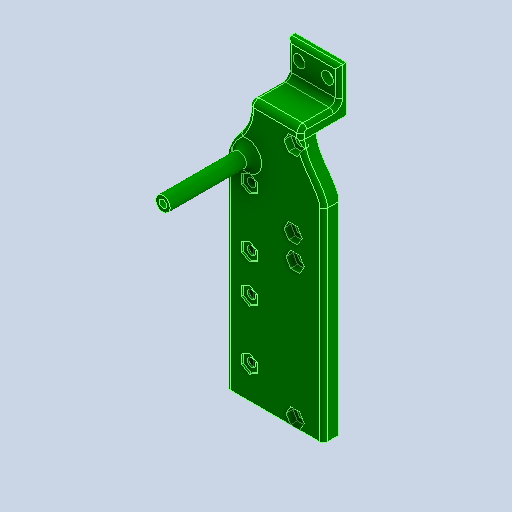
# Autodesk Inventor part: Battery_holder
Saved by Autodesk Inventor 2023.1 (Build 271208000, 208)
## iProperties
Created: 2022-08-12
Part Number: Battery_holder
Material: Default New Material
Document SubType Name: Modeling
Designer: Windows10
Density: 1 g/cm^3
Appearance: Generic
Author: Windows10
Autodesk Inventor part; units mm, degrees
ref_plane "YZ Plane" through (0, 0, 0) normal (1, 0, 0) x (0, 1, 0)
ref_plane "XZ Plane" through (0, 0, 0) normal (0, 1, 0) x (-1, 0, 0)
ref_plane "XY Plane" through (0, 0, 0) normal (0, 0, 1) x (1, 0, 0)
ref_plane "Work Plane2" through (3.3864, -46.8933, 3) normal (0, 0, 1) x (1, 0, 0)
sketch "Sketch1" plane through (3.3864, -46.8933, 3) normal (0, 0, 1) x (1, 0, 0)
  line L0 (-6.3864, -93.5067) -> (19.0636, -93.5067)
  line L1 (19.0636, -93.5067) -> (19.0636, -105.5067)
  line L2 (19.0636, -105.5067) -> (-6.3864, -105.5067)
  line L3 (-6.3864, -105.5067) -> (-6.3864, -93.5067)
  line L4 (-0.3864, -19.9067) -> (-0.3864, -27.9067) projected
  line L5 (-0.3864, -27.9067) -> (13.0636, -27.9067) projected
  line L6 (13.0636, -27.9067) -> (13.0636, -19.9067) projected
  line L7 (-0.3864, -27.9067) -> (-0.3864, -22.9067) projected
  line L8 (-0.3864, -27.9067) -> (13.0636, -27.9067)
  line L9 (13.0636, -27.9067) -> (13.0636, -15.9067)
  line L10 (13.0636, -15.9067) -> (-0.3864, -15.9067)
  line L11 (-0.3864, -15.9067) -> (-0.3864, -27.9067)
  point P0 (-3.3864, 46.8933)
  dimension "d1" = 25.45
  dimension "d2" = 12
  dimension "d3" = 13.45
  dimension "d4" = 12
  constraints: 16 end point, 4 parallel, 2 horizontal, 2 perpendicular
  measures "d1" distance of L1.end L2.end
  measures "d2" distance of L0.end L1.end
  measures "d3" distance of L10.end L9.end
  measures "d4" distance of L10.end L4.end
extrude "Extrusion1" add sketch "Sketch1" along normal blind 2
ref_plane "Work Plane3" through (3.3864, -46.8933, 5) normal (0, 0, 1) x (1, 0, 0)
sketch "Sketch2" plane through (3.3864, -46.8933, 5) normal (0, 0, 1) x (1, 0, 0)
  line L0 (19.0636, -93.5067) -> (-6.3864, -93.5067) projected
  line L1 (19.0636, -105.5067) -> (19.0636, -93.5067) projected
  line L2 (-6.3864, -93.5067) -> (19.0636, -93.5067)
  line L3 (19.0636, -93.5067) -> (19.0636, -96.5067)
  line L4 (19.0636, -96.5067) -> (-6.3864, -96.5067)
  line L5 (-6.3864, -96.5067) -> (-6.3864, -93.5067)
  line L6 (-0.3864, -27.9067) -> (-0.3864, -22.9067) projected
  line L7 (13.0636, -22.9067) -> (13.0636, -27.9067) projected
  line L8 (-0.3864, -27.9067) -> (13.0636, -27.9067)
  line L9 (13.0636, -27.9067) -> (13.0636, -24.9067)
  line L10 (13.0636, -24.9067) -> (-0.3864, -24.9067)
  line L11 (-0.3864, -24.9067) -> (-0.3864, -27.9067)
  point P0 (-3.3864, 46.8933)
  point P1 (-0.3864, -24.9067)
  dimension "d7" = 3
  dimension "d8" = 3
  constraints: 16 end point, 4 parallel, 2 horizontal, 2 perpendicular, 2 point on line
  measures "d7" distance of L2.end L3.end
  measures "d8" distance of L9.end L8.end
extrude "Extrusion2" add sketch "Sketch2" along normal blind 6
sketch "Sketch3" plane through (3.3864, -46.8933, 11) normal (0, 0, 1) x (1, 0, 0)
  line L0 (-6.3864, -96.5067) -> (19.0636, -96.5067) projected
  line L1 (19.0636, -96.5067) -> (19.0636, -93.5067) projected
  line L2 (19.0636, -93.5067) -> (-6.3864, -93.5067) projected
  line L3 (-6.3864, -93.5067) -> (-6.3864, -96.5067) projected
  line L4 (13.0636, -27.9067) -> (13.0636, -24.9067) projected
  line L5 (13.0636, -24.9067) -> (-0.3864, -24.9067) projected
  line L6 (-0.3864, -24.9067) -> (-0.3864, -27.9067) projected
  line L7 (-0.3864, -27.9067) -> (13.0636, -27.9067) projected
  line L8 (-6.3864, -96.5067) -> (19.0636, -96.5067)
  line L9 (19.0636, -96.5067) -> (19.0636, -40.4712)
  line L10 (19.0636, -40.4712) -> (-6.3864, -40.4712)
  line L11 (-6.3864, -40.4712) -> (-6.3864, -96.5067)
  line L12 (-6.3864, -40.4712) -> (-6.3864, -37.4338) construction
  line L13 (-6.3864, -37.4338) -> (-3.3864, -34.2758) construction
  line L14 (-3.3864, -34.2758) -> (-1.0738, -32.4773) construction
  line L15 (-1.0738, -32.4773) -> (-0.3864, -27.9067) construction
  spline S0 degree 4 poles (-6.3864, -40.4712) (-6.3864, -37.4338) (-3.3864, -34.2758) (-1.0738, -32.4773) (-0.3864, -27.9067) knots 1 1 1 1 1 2 2 2 2 2
  line L16 (6.3386, -40.4712) -> (6.3386, -46.7803)
  line L17 (19.0636, -40.4712) -> (19.0636, -37.4338) construction
  line L18 (19.0636, -37.4338) -> (16.0636, -34.2758) construction
  line L19 (16.0636, -34.2758) -> (13.7511, -32.4773) construction
  line L20 (13.7511, -32.4773) -> (13.0636, -27.9067) construction
  spline S1 degree 4 poles (19.0636, -40.4712) (19.0636, -37.4338) (16.0636, -34.2758) (13.7511, -32.4773) (13.0636, -27.9067) knots 1 1 1 1 1 2 2 2 2 2
  point P0 (-3.3864, 46.8933)
  point P1 (-6.3864, -93.5067)
  dimension "d11" = 25.45
  constraints: 10 end point, 3 symmetric about line, 2 parallel, 2 vertical, 1 horizontal, 1 midpoint, 1 perpendicular, 6 other
  measures "d11" distance of L10.end L9.end
extrude "Extrusion3" add sketch "Sketch3" along normal blind 4
sketch "Sketch4" plane through (3.3864, -46.8933, 5) normal (0, 0, 1) x (1, 0, 0)
  circle A0 centre (-1.3864, -101.5067) radius 1.75
  line L0 (-6.3864, -105.5067) -> (19.0636, -105.5067) projected
  line L1 (6.3386, -105.5067) -> (6.3386, -103.8916)
  line L2 (-6.3864, -96.5067) -> (-6.3864, -105.5067) projected
  line L3 (-6.3864, -96.5067) -> (19.0636, -96.5067) projected
  circle A1 centre (14.0636, -101.5067) radius 1.75
  circle A2 centre (2.6136, -19.9067) radius 1.5475
  line L4 (13.0636, -15.9067) -> (-0.3864, -15.9067) projected
  line L5 (6.3386, -15.9067) -> (6.3386, -14.3584)
  line L6 (-0.3864, -15.9067) -> (-0.3864, -24.9067) projected
  circle A3 centre (10.0636, -19.9067) radius 1.5475
  line L7 (13.0636, -24.9067) -> (-0.3864, -24.9067) projected
  point P0 (-3.3864, 46.8933)
  point P1 (-6.3864, -98.0067)
  dimension "d15" = 3.5
  dimension "d16" = 5
  dimension "d17" = 4
  dimension "d18" = 3
  dimension "d19" = 4
  dimension "d23" = 5
  dimension "d24" = 5
  dimension "d89" = 81.6
  dimension "d90" = 4
  dimension "d91" = 7.45
  dimension "d92" = 15.45
  dimension "d93" = 4
  constraints: 4 centre point, 4 end point, 2 midpoint, 2 symmetric about line, 2 vertical, 2 other
  measures "d15" diameter of A0
  measures "d16" distance from line of A0.centre L2
  measures "d17" distance from line of L0 A0.centre
  measures "d18" distance from line of L6 A2.centre
  measures "d19" distance from line of L4 A2.centre
  measures "d23" distance from line of L3 A0.centre
  measures "d24" distance from line of A2.centre L7
  measures "d89" vertical distance of A1.centre A3.centre
  measures "d90" horizontal distance of A3.centre A1.centre
  measures "d91" distance of A2.centre A3.centre
  measures "d92" distance of A0.centre A1.centre
  measures "d93" horizontal distance of A2.centre A0.centre
extrude "Extrusion4" cut sketch "Sketch4" against normal blind 2
fillet "Fillet2" radius 1.5 4 edges at (9.725, -143.4, 15) (9.725, -143.4, 5) (9.725, -71.8, 15) (9.725, -71.8, 5)
sketch "Sketch6" plane through (3.3864, -46.8933, 15) normal (0, 0, 1) x (1, 0, 0)
  line L0 (9.0398, -52.206) -> (21.0398, -52.206)
  line L1 (21.0398, -52.206) -> (21.0398, -27.206)
  line L2 (21.0398, -27.206) -> (9.0398, -27.206)
  line L3 (9.0398, -27.206) -> (9.0398, -52.206)
  line L4 (9.0398, -93.9784) -> (29.3398, -93.9784)
  line L5 (29.3398, -93.9784) -> (29.3398, -53.3784)
  line L6 (29.3398, -53.3784) -> (9.0398, -53.3784)
  line L7 (9.0398, -53.3784) -> (9.0398, -93.9784)
  circle A0 centre (11.0398, -29.706) radius 1.1
  circle A1 centre (11.5798, -91.4384) radius 1.1
  line L8 (9.0398, -73.6784) -> (6.4211, -73.6784)
  circle A2 centre (11.5798, -55.9184) radius 1.1
  line L9 (12.7648, -89.3859) -> (13.9498, -91.4384)
  line L10 (13.9498, -91.4384) -> (12.7648, -93.4909)
  line L11 (12.7648, -93.4909) -> (10.3948, -93.4909)
  line L12 (10.3948, -93.4909) -> (9.2098, -91.4384)
  line L13 (9.2098, -91.4384) -> (10.3948, -89.3859)
  line L14 (10.3948, -89.3859) -> (12.7648, -89.3859)
  circle A3 centre (11.5798, -91.4384) radius 3.5
  circle A4 centre (11.5798, -55.9184) radius 1.1
  line L15 (12.7648, -57.9709) -> (13.9498, -55.9184)
  line L16 (13.9498, -55.9184) -> (12.7648, -53.8659)
  line L17 (12.7648, -53.8659) -> (10.3948, -53.8659)
  line L18 (10.3948, -53.8659) -> (9.2098, -55.9184)
  line L19 (9.2098, -55.9184) -> (10.3948, -57.9709)
  line L20 (10.3948, -57.9709) -> (12.7648, -57.9709)
  circle A5 centre (11.5798, -55.9184) radius 3.5
  circle A6 centre (11.0398, -29.706) radius 1.1
  line L21 (9.8548, -31.7585) -> (12.2248, -31.7585)
  line L22 (8.6698, -29.706) -> (9.8548, -31.7585)
  line L23 (12.2248, -31.7585) -> (13.4098, -29.706)
  circle A7 centre (11.0398, -29.706) radius 1.1
  line L24 (13.4098, -29.706) -> (12.2248, -27.6536)
  line L25 (12.2248, -27.6536) -> (9.8548, -27.6536)
  line L26 (9.8548, -27.6536) -> (8.6698, -29.706)
  circle A8 centre (11.0398, -29.706) radius 3.5
  line L27 (-0.3864, -26.4067) -> (13.0636, -26.4067) projected
  line L28 (6.3386, -26.4067) -> (6.3386, -33.206)
  line L29 (3.6375, -27.206) -> (3.6375, -52.206)
  circle A9 centre (1.6375, -29.706) radius 1.1
  line L30 (4.0075, -29.706) -> (2.8225, -31.7585)
  line L31 (2.8225, -31.7585) -> (0.4525, -31.7585)
  line L32 (0.4525, -27.6536) -> (2.8225, -27.6536)
  line L33 (-0.7325, -29.706) -> (0.4525, -27.6536)
  line L34 (2.8225, -27.6536) -> (4.0075, -29.706)
  line L35 (0.4525, -31.7585) -> (-0.7325, -29.706)
  line L36 (13.0636, -23.4067) -> (-0.3864, -23.4067) projected
  line L37 (9.0398, -39.706) -> (7.6363, -39.706)
  circle A10 centre (11.0398, -49.706) radius 1.1
  line L38 (8.6698, -49.706) -> (9.8548, -47.6536)
  line L39 (9.8548, -47.6536) -> (12.2248, -47.6536)
  line L40 (12.2248, -51.7585) -> (9.8548, -51.7585)
  line L41 (13.4098, -49.706) -> (12.2248, -51.7585)
  line L42 (9.8548, -51.7585) -> (8.6698, -49.706)
  line L43 (12.2248, -47.6536) -> (13.4098, -49.706)
  circle A11 centre (-0.3864, -85.0067) radius 1.1
  line L44 (-6.3864, -40.4712) -> (-6.3864, -95.0067) projected
  line L45 (-0.3864, -85.0067) -> (-0.3864, -77.2817)
  line L46 (-0.3864, -77.2817) -> (0.7136, -77.2817)
  line L47 (-0.3864, -87.3767) -> (-2.4389, -86.1917)
  line L48 (-2.4389, -86.1917) -> (-2.4389, -83.8217)
  line L49 (-2.4389, -83.8217) -> (-0.3864, -82.6366)
  line L50 (-0.3864, -82.6366) -> (1.6661, -83.8217)
  line L51 (1.6661, -83.8217) -> (1.6661, -86.1917)
  line L52 (1.6661, -86.1917) -> (-0.3864, -87.3767)
  circle A12 centre (-0.3864, -69.5567) radius 1.1
  line L53 (-0.3864, -67.1866) -> (-2.4389, -68.3717)
  line L54 (-2.4389, -68.3717) -> (-2.4389, -70.7417)
  line L55 (-2.4389, -70.7417) -> (-0.3864, -71.9267)
  line L56 (-0.3864, -71.9267) -> (1.6661, -70.7417)
  line L57 (1.6661, -70.7417) -> (1.6661, -68.3717)
  line L58 (1.6661, -68.3717) -> (-0.3864, -67.1866)
  line L59 (9.0398, -64.5567) -> (-9.8125, -64.5567)
  circle A13 centre (-0.3864, -44.1067) radius 1.1
  line L60 (-0.3864, -44.1067) -> (-0.3864, -51.8317)
  line L61 (-0.3864, -51.8317) -> (0.7136, -51.8317)
  line L62 (-0.3864, -41.7366) -> (-2.4389, -42.9217)
  line L63 (-2.4389, -42.9217) -> (-2.4389, -45.2917)
  line L64 (-2.4389, -45.2917) -> (-0.3864, -46.4767)
  line L65 (-0.3864, -46.4767) -> (1.6661, -45.2917)
  line L66 (1.6661, -45.2917) -> (1.6661, -42.9217)
  line L67 (1.6661, -42.9217) -> (-0.3864, -41.7366)
  line L68 (-2.4389, -60.7417) -> (-2.4389, -58.3717)
  circle A14 centre (-0.3864, -59.5567) radius 1.1
  line L69 (-0.3864, -57.1866) -> (1.6661, -58.3717)
  line L70 (1.6661, -58.3717) -> (1.6661, -60.7417)
  line L71 (1.6661, -60.7417) -> (-0.3864, -61.9267)
  line L72 (-0.3864, -61.9267) -> (-2.4389, -60.7417)
  line L73 (-2.4389, -58.3717) -> (-0.3864, -57.1866)
  line L74 (-3.4389, -83.2443) -> (-3.4389, -86.769)
  line L75 (-3.4389, -86.769) -> (-0.3864, -88.5314)
  line L76 (-0.3864, -88.5314) -> (2.6661, -86.769)
  line L77 (2.6661, -86.769) -> (2.6661, -83.2443)
  line L78 (2.6661, -83.2443) -> (-0.3864, -81.4819)
  line L79 (-0.3864, -81.4819) -> (-3.4389, -83.2443)
  line L80 (-3.4389, -71.319) -> (-3.4389, -67.7943)
  line L81 (-3.4389, -67.7943) -> (-0.3864, -66.0319)
  line L82 (-0.3864, -66.0319) -> (2.6661, -67.7943)
  line L83 (2.6661, -67.7943) -> (2.6661, -71.319)
  line L84 (2.6661, -71.319) -> (-0.3864, -73.0814)
  line L85 (-0.3864, -73.0814) -> (-3.4389, -71.319)
  line L86 (-3.4389, -57.7943) -> (-3.4389, -61.319)
  line L87 (-3.4389, -61.319) -> (-0.3864, -63.0814)
  line L88 (-0.3864, -63.0814) -> (2.6661, -61.319)
  line L89 (2.6661, -61.319) -> (2.6661, -57.7943)
  line L90 (2.6661, -57.7943) -> (-0.3864, -56.0319)
  line L91 (-0.3864, -56.0319) -> (-3.4389, -57.7943)
  line L92 (-3.4389, -42.3443) -> (-0.3864, -40.5819)
  line L93 (-0.3864, -40.5819) -> (2.6661, -42.3443)
  line L94 (2.6661, -42.3443) -> (2.6661, -45.869)
  line L95 (2.6661, -45.869) -> (-0.3864, -47.6314)
  line L96 (-0.3864, -47.6314) -> (-3.4389, -45.869)
  line L97 (-3.4389, -45.869) -> (-3.4389, -42.3443)
  point P0 (-3.3864, 46.8933)
  point P1 (15.0398, -52.206)
  point P2 (8.4998, -46.166)
  point P3 (8.4998, -27.166)
  point P4 (-6.3864, -96.5067)
  point P5 (-0.3864, -64.5567)
  point P6 (6.4211, -55.4349)
  dimension "d47" = 12
  dimension "d48" = 25
  dimension "d49" = 20.3
  dimension "d50" = 40.6
  dimension "d54" = 2.2
  dimension "d55" = 2
  dimension "d56" = 2.5
  dimension "d57" = 2.2
  dimension "d58" = 2.54
  dimension "d59" = 2.54
  dimension "d60" = 4.74
  dimension "d61" = 7
  dimension "d99" = 4.2469
  dimension "d100" = 2.54
  dimension "d101" = 2.2
  dimension "d102" = 6
  dimension "d103" = 4.105
  dimension "d104" = 11.5
  dimension "d105" = 7.725
  dimension "d106" = 4.105
  dimension "d107" = 5
  dimension "d108" = 1
  dimension "d109" = 1
  dimension "d110" = 1
  dimension "d111" = 1
  constraints: 190 end point, 53 symmetric about line, 15 centre point, 7 coincident, 6 horizontal, 5 midpoint, 4 parallel, 2 perpendicular, 2 vertical, 1 collinear, 1 point on line, 54 other
  measures "d47" distance of L2.end L1.end
  measures "d48" distance of L1.end L0.end
  measures "d49" distance of L6.end L5.end
  measures "d50" distance of L5.end L4.end
  measures "d54" diameter of A0
  measures "d55" distance from line of A0.centre L3
  measures "d56" distance from line of L2 A0.centre
  measures "d57" diameter of A1
  measures "d58" distance from line of L7 A1.centre
  measures "d59" distance from line of L4 A1.centre
  measures "d60" distance of L9.end L12.end
  measures "d61" diameter of A3
  measures "d99" distance between parallel lines of L36 L25
  measures "d100" distance from line of L7 A5.centre
  measures "d101" diameter of A11
  measures "d102" distance from line of L44 L45.start
  measures "d103" distance between parallel lines of L14 L11
  measures "d104" vertical distance of point (-6.386, -96.507) L45.start
  measures "d105" distance of L45.start L45.end
  measures "d106" distance between parallel lines of L51 L48
  measures "d107" distance of A12.centre point (-0.386, -64.557)
  measures "d108" distance between parallel lines of L48 L74
  measures "d109" distance between parallel lines of L54 L80
  measures "d110" distance between parallel lines of L68 L86
  measures "d111" distance between parallel lines of L62 L92
extrude "Extrusion5" cut sketch "Sketch6" against normal blind 1.8 contours L42 L38 L3 | L3 L38 L39 L43 L41 L40 L42 | L26 L25 L24 L23 L21 L22 L3 | L3 L22 L26 | A0 | A1 | A2 | L9 L10 L11 L12 L13 L14 | L20 L19 L18 L17 L16 L15 | A10
ref_plane "Work Plane4" through (-3, -140.4, 3) normal (0, 1, 0) x (1, 0, 0)
split body "Split1" result two bodies by plane through (-3, -140.4, 3) normal (0, 1, 0) first body at (13.9667, -122.7215, 11.5)
sketch "Sketch7" plane through (-3, -140.4, 15) normal (0, -1, 0) x (1, 0, 0)
  line L0 (14.45, -1) -> (4, -1)
  line L1 (4, -1) -> (4, -3)
  line L2 (4, -3) -> (14.45, -3)
  line L3 (14.45, -3) -> (14.45, -1)
  line L4 (25.45, -4) -> (25.45, 0) projected
  line L5 (0, 0) -> (0, -4) projected
  line L6 (25.45, -4) -> (0, -4) projected
  line L7 (25.45, 0) -> (0, 0) projected
  point P0 (3, -15)
  point P1 (15.5961, 0)
  point P2 (25.45, -2)
  dimension "d65" = 11
  dimension "d66" = 4
  dimension "d67" = 2
  dimension "d69" = 1
  dimension "d70" = 1
  constraints: 8 end point, 2 parallel, 1 horizontal, 1 midpoint, 1 perpendicular
  measures "d65" distance from line of point (25.45, -2) L3
  measures "d66" distance between parallel lines of L5 L1
  measures "d67" distance of L0.end L1.end
  measures "d69" distance between parallel lines of L7 L0
  measures "d70" distance between parallel lines of L6 L2
extrude "Extrusion6" cut sketch "Sketch7" against normal blind 48 contours L3 L2 L1 L0 bodies 2
sketch "Sketch8" plane through (-3, -140.4, 3) normal (0, 1, 0) x (1, 0, 0)
  line L0 (14.45, -1.1) -> (4, -1.1)
  line L1 (4, -1.1) -> (4, -2.9)
  line L2 (4, -2.9) -> (14.45, -2.9)
  line L3 (14.45, -2.9) -> (14.45, -1.1)
  line L4 (25.45, -4) -> (25.45, 0)
  line L5 (0, 0) -> (0, -4)
  line L6 (25.45, -4) -> (0, -4)
  line L7 (25.45, 0) -> (0, 0)
  line L8 (30.2309, -12) -> (30.2309, 0)
  line L9 (30.2309, -6) -> (31.8513, -6)
  line L10 (14.45, -10.9) -> (4, -10.9)
  line L11 (4, -10.9) -> (4, -9.1)
  line L12 (4, -9.1) -> (14.45, -9.1)
  line L13 (14.45, -9.1) -> (14.45, -10.9)
  line L14 (25.45, -8) -> (25.45, -12)
  line L15 (0, -12) -> (0, -8)
  line L16 (25.45, -8) -> (0, -8)
  line L17 (25.45, -12) -> (0, -12)
  line L18 (4.3, -10.6) -> (14.15, -10.6)
  line L19 (14.15, -10.6) -> (14.15, -9.4)
  line L20 (14.15, -9.4) -> (4.3, -9.4)
  line L21 (4.3, -9.4) -> (4.3, -10.6)
  point P0 (3, 3)
  point P1 (3, -15)
  point P2 (15.5961, 0)
  point P3 (25.45, -2)
  point P4 (15.5961, -12)
  point P5 (25.45, -10)
  dimension "d73" = 11
  dimension "d74" = 4
  dimension "d75" = 1.8
  dimension "d76" = 1.1
  dimension "d77" = 1.1
  dimension "d78" = 0.3
  constraints: 44 end point, 10 symmetric about line, 2 horizontal, 2 midpoint, 2 parallel, 1 perpendicular, 1 vertical, 3 other
  measures "d73" distance from line of point (25.45, -2) L3
  measures "d74" distance between parallel lines of L5 L1
  measures "d75" distance of L0.end L1.end
  measures "d76" distance between parallel lines of L7 L0
  measures "d77" distance between parallel lines of L6 L2
  measures "d78" distance between parallel lines of L10 L18
extrude "Extrusion7" add sketch "Sketch8" along normal blind 48 contours L21 L20 L19 L18 bodies 3
sketch "Sketch9" plane through (3.3864, -46.8933, 15) normal (0, 0, 1) x (1, 0, 0)
  line L0 (-1.0605, -90.0613) -> (-1.0605, -38.0613)
  circle A0 centre (-1.0605, -90.0613) radius 1
  circle A1 centre (-1.0605, -38.0613) radius 1
  circle A2 centre (-1.0605, -90.0613) radius 1.9
  circle A3 centre (-1.0605, -38.0613) radius 1.9
  line L1 (19.0636, -93.5067) -> (-6.3864, -93.5067) projected
  point P0 (-3.3864, 46.8933)
  point P1 (-3.3864, 46.8933)
  dimension "d81" = 52
  dimension "d82" = 2
  dimension "d83" = 2
  dimension "d84" = 3.8
  dimension "d85" = 3.8
  dimension "d150" = 3.4453
  constraints: 4 centre point, 4 coincident, 2 end point, 1 vertical
  measures "d81" distance of L0.start L0.end
  measures "d82" diameter of A0
  measures "d83" diameter of A1
  measures "d84" diameter of A2
  measures "d85" diameter of A3
  measures "d150" distance from line of L1 L0.start
extrude "Extrusion8" add sketch "Sketch9" along normal blind 22 contours A3 bodies 2
fillet "Fillet3" radius 2 1 edges at (0.4258, -84.9547, 15)
extrude "Extrusion9" cut sketch "Sketch6" against normal blind 12.25 contours A0 | A1 | A2 | A10 bodies 2
extrude "Extrusion10" [suppressed]
sketch "Sketch11" plane through (3.3864, -46.8933, 16.5) normal (0, 0, 1) x (1, 0, 0)
  line L0 (9.0398, -52.206) -> (21.0398, -52.206)
  line L1 (21.0398, -52.206) -> (21.0398, -27.206)
  line L2 (21.0398, -27.206) -> (9.0398, -27.206)
  line L3 (9.0398, -27.206) -> (9.0398, -52.206)
  line L4 (9.0398, -93.9784) -> (29.3398, -93.9784)
  line L5 (29.3398, -93.9784) -> (29.3398, -53.3784)
  line L6 (29.3398, -53.3784) -> (9.0398, -53.3784)
  line L7 (9.0398, -53.3784) -> (9.0398, -93.9784)
  circle A0 centre (11.0398, -29.706) radius 1.1
  circle A1 centre (11.5798, -91.4384) radius 1.1
  line L8 (9.0398, -73.6784) -> (6.4211, -73.6784)
  circle A2 centre (11.5798, -55.9184) radius 1.1
  line L9 (12.7648, -89.3859) -> (13.9498, -91.4384)
  line L10 (13.9498, -91.4384) -> (12.7648, -93.4909)
  line L11 (12.7648, -93.4909) -> (10.3948, -93.4909)
  line L12 (10.3948, -93.4909) -> (9.2098, -91.4384)
  line L13 (9.2098, -91.4384) -> (10.3948, -89.3859)
  line L14 (10.3948, -89.3859) -> (12.7648, -89.3859)
  circle A3 centre (11.5798, -91.4384) radius 3.5
  line L15 (10.3948, -57.9709) -> (12.7648, -57.9709)
  line L16 (9.2098, -55.9184) -> (10.3948, -57.9709)
  line L17 (12.7648, -57.9709) -> (13.9498, -55.9184)
  circle A4 centre (11.5798, -55.9184) radius 1.1
  line L18 (13.9498, -55.9184) -> (12.7648, -53.8659)
  line L19 (12.7648, -53.8659) -> (10.3948, -53.8659)
  line L20 (10.3948, -53.8659) -> (9.2098, -55.9184)
  circle A5 centre (11.5798, -55.9184) radius 3.5
  line L21 (8.6698, -29.706) -> (9.8548, -31.7585)
  line L22 (9.8548, -31.7585) -> (12.2248, -31.7585)
  circle A6 centre (11.0398, -29.706) radius 3.5
  circle A7 centre (11.0398, -29.706) radius 1.1
  line L23 (12.2248, -27.6536) -> (9.8548, -27.6536)
  line L24 (13.4098, -29.706) -> (12.2248, -27.6536)
  line L25 (9.8548, -27.6536) -> (8.6698, -29.706)
  circle A8 centre (11.0398, -29.706) radius 1.1
  line L26 (12.2248, -31.7585) -> (13.4098, -29.706)
  line L27 (-0.3864, -26.4067) -> (13.0636, -26.4067)
  line L28 (6.3386, -26.4067) -> (6.3386, -33.206)
  line L29 (4.0075, -29.706) -> (2.8225, -31.7585)
  line L30 (3.6375, -27.206) -> (3.6375, -52.206)
  line L31 (0.4525, -27.6536) -> (2.8225, -27.6536)
  line L32 (-0.7325, -29.706) -> (0.4525, -27.6536)
  line L33 (0.4525, -31.7585) -> (-0.7325, -29.706)
  line L34 (2.8225, -31.7585) -> (0.4525, -31.7585)
  circle A9 centre (1.6375, -29.706) radius 1.1
  line L35 (2.8225, -27.6536) -> (4.0075, -29.706)
  line L36 (13.0636, -23.4067) -> (-0.3864, -23.4067)
  line L37 (9.0398, -39.706) -> (7.6363, -39.706)
  line L38 (9.8548, -51.7585) -> (8.6698, -49.706)
  line L39 (8.6698, -49.706) -> (9.8548, -47.6536)
  line L40 (9.8548, -47.6536) -> (12.2248, -47.6536)
  line L41 (12.2248, -47.6536) -> (13.4098, -49.706)
  line L42 (13.4098, -49.706) -> (12.2248, -51.7585)
  line L43 (12.2248, -51.7585) -> (9.8548, -51.7585)
  circle A10 centre (11.0398, -49.706) radius 1.1
  circle A11 centre (-0.3864, -85.0067) radius 1.1
  line L44 (-10.3864, -40.4712) -> (-10.3864, -95.0067)
  line L45 (-0.3864, -85.0067) -> (-0.3864, -77.2817)
  line L46 (-0.3864, -77.2817) -> (0.7136, -77.2817)
  line L47 (-0.3864, -87.3767) -> (-2.4389, -86.1917)
  line L48 (-2.4389, -86.1917) -> (-2.4389, -83.8217)
  line L49 (-2.4389, -83.8217) -> (-0.3864, -82.6366)
  line L50 (-0.3864, -82.6366) -> (1.6661, -83.8217)
  line L51 (1.6661, -83.8217) -> (1.6661, -86.1917)
  line L52 (1.6661, -86.1917) -> (-0.3864, -87.3767)
  line L53 (-2.4389, -68.3717) -> (-2.4389, -70.7417)
  circle A12 centre (-0.3864, -69.5567) radius 1.1
  line L54 (-0.3864, -71.9267) -> (1.6661, -70.7417)
  line L55 (1.6661, -70.7417) -> (1.6661, -68.3717)
  line L56 (1.6661, -68.3717) -> (-0.3864, -67.1866)
  line L57 (-0.3864, -67.1866) -> (-2.4389, -68.3717)
  line L58 (-2.4389, -70.7417) -> (-0.3864, -71.9267)
  line L59 (9.0398, -64.5567) -> (-9.8125, -64.5567)
  line L60 (-0.3864, -51.8317) -> (0.7136, -51.8317)
  line L61 (-0.3864, -46.4767) -> (1.6661, -45.2917)
  line L62 (-2.4389, -45.2917) -> (-0.3864, -46.4767)
  line L63 (-0.3864, -44.1067) -> (-0.3864, -51.8317)
  circle A13 centre (-0.3864, -44.1067) radius 1.1
  line L64 (1.6661, -45.2917) -> (1.6661, -42.9217)
  line L65 (-2.4389, -42.9217) -> (-2.4389, -45.2917)
  line L66 (1.6661, -42.9217) -> (-0.3864, -41.7366)
  line L67 (-0.3864, -41.7366) -> (-2.4389, -42.9217)
  line L68 (-0.3864, -57.1866) -> (1.6661, -58.3717)
  line L69 (-2.4389, -58.3717) -> (-0.3864, -57.1866)
  circle A14 centre (-0.3864, -59.5567) radius 1.1
  line L70 (1.6661, -58.3717) -> (1.6661, -60.7417)
  line L71 (-2.4389, -60.7417) -> (-2.4389, -58.3717)
  line L72 (1.6661, -60.7417) -> (-0.3864, -61.9267)
  line L73 (-0.3864, -61.9267) -> (-2.4389, -60.7417)
  line L74 (-3.4389, -83.2443) -> (-3.4389, -86.769)
  line L75 (-3.4389, -86.769) -> (-0.3864, -88.5314)
  line L76 (-0.3864, -88.5314) -> (2.6661, -86.769)
  line L77 (2.6661, -86.769) -> (2.6661, -83.2443)
  line L78 (2.6661, -83.2443) -> (-0.3864, -81.4819)
  line L79 (-0.3864, -81.4819) -> (-3.4389, -83.2443)
  line L80 (-3.4389, -71.319) -> (-3.4389, -67.7943)
  line L81 (-3.4389, -67.7943) -> (-0.3864, -66.0319)
  line L82 (-0.3864, -66.0319) -> (2.6661, -67.7943)
  line L83 (2.6661, -67.7943) -> (2.6661, -71.319)
  line L84 (2.6661, -71.319) -> (-0.3864, -73.0814)
  line L85 (-0.3864, -73.0814) -> (-3.4389, -71.319)
  line L86 (-3.4389, -57.7943) -> (-3.4389, -61.319)
  line L87 (-3.4389, -61.319) -> (-0.3864, -63.0814)
  line L88 (-0.3864, -63.0814) -> (2.6661, -61.319)
  line L89 (2.6661, -61.319) -> (2.6661, -57.7943)
  line L90 (2.6661, -57.7943) -> (-0.3864, -56.0319)
  line L91 (-0.3864, -56.0319) -> (-3.4389, -57.7943)
  line L92 (-3.4389, -42.3443) -> (-0.3864, -40.5819)
  line L93 (-0.3864, -40.5819) -> (2.6661, -42.3443)
  line L94 (2.6661, -42.3443) -> (2.6661, -45.869)
  line L95 (2.6661, -45.869) -> (-0.3864, -47.6314)
  line L96 (-0.3864, -47.6314) -> (-3.4389, -45.869)
  line L97 (-3.4389, -45.869) -> (-3.4389, -42.3443)
  line L98 (19.0636, -95.0067) -> (-6.3864, -95.0067) projected
  point P0 (-3.3864, 46.8933)
  point P1 (-3.3864, 46.8933)
  point P2 (15.0398, -52.206)
  point P3 (8.4998, -46.166)
  point P4 (8.4998, -27.166)
  point P5 (-10.3864, -93.5067)
  point P6 (-0.3864, -64.5567)
  point P7 (6.4211, -55.4349)
  dimension "d114" = 12
  dimension "d115" = 25
  dimension "d116" = 20.3
  dimension "d117" = 40.6
  dimension "d118" = 2.2
  dimension "d119" = 2
  dimension "d120" = 2.5
  dimension "d121" = 2.2
  dimension "d122" = 2.54
  dimension "d123" = 2.54
  dimension "d124" = 4.74
  dimension "d125" = 7
  dimension "d126" = 4.2469
  dimension "d127" = 2.54
  dimension "d128" = 2.2
  dimension "d129" = 10
  dimension "d130" = 4.105
  dimension "d131" = 8.5
  dimension "d132" = 7.725
  dimension "d133" = 4.105
  dimension "d134" = 5
  dimension "d135" = 1
  dimension "d136" = 1
  dimension "d137" = 1
  dimension "d138" = 1
  dimension "d144" = 9.4261
  dimension "d145" = 10
  constraints: 196 end point, 53 symmetric about line, 15 centre point, 7 coincident, 6 horizontal, 5 midpoint, 4 parallel, 2 perpendicular, 2 vertical, 1 collinear, 1 point on line, 54 other
  measures "d114" distance of L2.end L1.end
  measures "d115" distance of L1.end L0.end
  measures "d116" distance of L6.end L5.end
  measures "d117" distance of L5.end L4.end
  measures "d118" diameter of A0
  measures "d119" distance from line of A0.centre L3
  measures "d120" distance from line of L2 A0.centre
  measures "d121" diameter of A1
  measures "d122" distance from line of L7 A1.centre
  measures "d123" distance from line of L4 A1.centre
  measures "d124" distance of L9.end L12.end
  measures "d125" diameter of A3
  measures "d126" distance between parallel lines of L36 L23
  measures "d127" distance from line of L7 A5.centre
  measures "d128" diameter of A11
  measures "d129" distance from line of L44 L45.start
  measures "d130" distance between parallel lines of L14 L11
  measures "d131" vertical distance of point (-10.386, -93.507) L45.start
  measures "d132" distance of L45.start L45.end
  measures "d133" distance between parallel lines of L51 L48
  measures "d134" distance of A12.centre point (-0.386, -64.557)
  measures "d135" distance between parallel lines of L48 L74
  measures "d136" distance between parallel lines of L53 L80
  measures "d137" distance between parallel lines of L71 L86
  measures "d138" distance between parallel lines of L67 L92
  measures "d144" distance from line of L7 L45.start
  measures "d145" distance from line of L98 L45.start
extrude "Extrusion11" [suppressed]
extrude "Extrusion12" [suppressed]
fillet "Fillet4" radius 1 26 edges at (19.6219, -81.4982, 15) (22.45, -113.8823, 15) (-0.1719, -81.4982, 15) (-3, -113.8823, 15) (16.45, -72.2393, 14.5607) (16.45, -74.05, 15) (16.45, -71.3607, 5.4393) (16.45, -66.55, 5) (16.45, -71.8, 10) (3, -74.05, 15) (3, -71.8, 10) (3, -71.3607, 5.4393) (3, -66.55, 5) (3, -72.2393, 14.5607) (9.725, -62.8, 5) (9.725, -152.4, 5) (22.45, -143.8393, 5.4393) (22.45, -143.4, 10) (22.45, -142.9607, 14.5607) (22.45, -141.15, 15) (22.45, -148.65, 5) (-3, -143.8393, 5.4393) (-3, -143.4, 10) (-3, -142.9607, 14.5607) (-3, -141.15, 15) (-3, -148.65, 5)
extrude "Extrusion13" cut sketch "Sketch6" along normal blind 1 and the other way blind 0.5 contours A11 | L47 L48 L49 L50 L51 L52 | A12 | L58 L57 L56 L55 L54 L53 | A13 | L67 L66 L65 L64 L63 L62 | L68 L73 L69 L70 L71 L72 | A14 bodies 2
extrude "Extrusion14" cut sketch "Sketch6" against normal blind 3 contours A11 | A12 | A13 | A14 bodies 2
body "Solid3"
body "Solid4"
